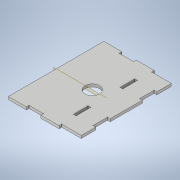
# Autodesk Inventor part: Side_two
Saved by Autodesk Inventor 2020 (Build 240168000, 168)
## iProperties
Created: 2019-12-17
Part Number: Side_two
Material: Generic
Document SubType Name: Modeling
Designer: fabfarm
Density: 1 g/cm^3
Appearance: Default
Author: fabfarm
Autodesk Inventor part; units mm, degrees
ref_plane "YZ Plane" through (0, 0, 0) normal (1, 0, 0) x (0, 1, 0)
ref_plane "XZ Plane" through (0, 0, 0) normal (0, 1, 0) x (-1, 0, 0)
ref_plane "XY Plane" through (0, 0, 0) normal (0, 0, 1) x (1, 0, 0)
sketch "Sketch1" plane through (0, 0, 0) normal (0, 1, 0) x (-1, 0, 0)
  line L0 (0, 0) -> (485, 0)
  line L1 (485, 0) -> (485, 660)
  line L2 (485, 660) -> (0, 660)
  line L3 (0, 660) -> (0, 0)
  dimension "d0" = 485
  dimension "d1" = 660
  constraints: 8 end point, 2 parallel, 1 horizontal, 1 perpendicular
  measures "d0" distance of L0.start L0.end
  measures "d1" distance of L2.end L0.start
extrude "Extrusion1" add sketch "Sketch1" along normal blind 18.55
ref_plane "Work Plane1" through (-485, 0, 330) normal (0, 0, 1) x (1, 0, 0)
sketch "Sketch4" plane through (0, 18.55, 0) normal (0, 1, 0) x (1, 0, 0)
  circle A0 centre (-235, -330) radius 50
  line L0 (97, -330) -> (-582, -330) projected
  line L1 (0, -660) -> (0, 0) projected
  point P0 (0, -641.45)
  point P1 (0, -18.55)
  dimension "d20" = 100
  dimension "d21" = 235
  constraints: 1 centre point, 1 point on line
  measures "d20" diameter of A0
  measures "d21" distance from line of L1 A0.centre
extrude "Extrusion4" cut sketch "Sketch4" against normal blind 20
sketch "Esquisse5" plane through (0, 18.55, 0) normal (0, 1, 0) x (1, 0, 0)
  line L0 (-485, -660) -> (0, -660) projected
  line L1 (-360.1, -660) -> (-259.9, -660)
  line L2 (-259.9, -660) -> (-259.9, -641.45)
  line L3 (-259.9, -641.45) -> (-360.1, -641.45)
  line L4 (-360.1, -641.45) -> (-360.1, -660)
  line L5 (0, 0) -> (-485, 0) projected
  line L6 (-360.1, 0) -> (-259.9, 0)
  line L7 (-259.9, 0) -> (-259.9, -18.55)
  line L8 (-259.9, -18.55) -> (-360.1, -18.55)
  line L9 (-360.1, -18.55) -> (-360.1, 0)
  line L10 (-485, 0) -> (-485, -660) projected
  line L11 (0, -660) -> (0, 0) projected
  point P0 (-259.9, -660)
  dimension "d24" = 100.2
  dimension "d25" = 124.9
  dimension "d26" = 18.55
  dimension "d27" = 18.55
  dimension "d28" = 259.9
  constraints: 16 end point, 4 parallel, 4 point on line, 2 horizontal, 2 perpendicular
  measures "d24" distance of L2.end L3.end
  measures "d25" distance between parallel lines of L10 L4
  measures "d26" distance of L1.end L2.end
  measures "d27" distance of L6.end L7.end
  measures "d28" distance from line of L11 L1.end
extrude "Extrusion5" cut sketch "Esquisse5" against normal blind 100 contours L4 L3 L2 L0 | L5 L7 L8 L9
sketch "Esquisse6" plane through (0, 18.55, 0) normal (0, 1, 0) x (1, 0, 0)
  line L0 (-259.9, -18.55) -> (-360.1, -18.55) projected
  circle A0 centre (-360.1, -18.55) radius 1.585
  circle A1 centre (-259.9, -18.55) radius 1.585
  line L1 (-259.9, -641.45) -> (-360.1, -641.45) projected
  circle A2 centre (-360.1, -641.45) radius 1.585
  circle A3 centre (-259.9, -641.45) radius 1.585
  point P0 (0, 0)
  dimension "d31" = 3.17
  constraints: 4 centre point, 3 equal radius, 2 coincident
  measures "d31" diameter of A3
extrude "Extrusion6" cut sketch "Esquisse6" against normal blind 100
sketch "Esquisse7" plane through (0, 18.55, 0) normal (0, 1, 0) x (1, 0, 0)
  line L0 (-134.85, -541.5) -> (-153.5, -541.5)
  line L1 (-153.5, -541.5) -> (-153.5, -441.4)
  line L2 (-153.5, -441.4) -> (-134.85, -441.4)
  line L3 (-134.85, -441.4) -> (-134.85, -541.5)
  line L4 (-134.85, -218.6) -> (-153.5, -218.6)
  line L5 (-153.5, -218.6) -> (-153.5, -118.5)
  line L6 (-153.5, -118.5) -> (-134.85, -118.5)
  line L7 (-134.85, -118.5) -> (-134.85, -218.6)
  line L8 (0, 0) -> (-259.9, 0) projected
  line L9 (-259.9, -660) -> (0, -660) projected
  line L10 (-259.9, -643.035) -> (-259.9, -660) projected
  dimension "d34" = 118.5
  dimension "d35" = 100.1
  dimension "d36" = 100.1
  dimension "d37" = 118.5
  dimension "d38" = 18.65
  dimension "d45" = 106.4
  constraints: 16 end point, 4 parallel, 2 collinear, 2 horizontal, 2 perpendicular
  measures "d34" distance between parallel lines of L8 L6
  measures "d35" distance of L4.end L5.end
  measures "d36" distance of L0.end L1.end
  measures "d37" distance between parallel lines of L9 L0
  measures "d38" distance of L1.end L2.end
  measures "d45" distance between parallel lines of L10 L1
extrude "Extrusion7" cut sketch "Esquisse7" against normal blind 20
sketch "Esquisse8" plane through (0, 18.55, 0) normal (0, 1, 0) x (1, 0, 0)
  line L0 (-153.5, -541.5) -> (-153.5, -441.4) projected
  circle A0 centre (-153.5, -541.5) radius 1.6
  circle A1 centre (-153.5, -441.4) radius 1.6
  line L1 (-153.5, -218.6) -> (-153.5, -118.5) projected
  circle A2 centre (-153.5, -218.6) radius 1.6
  circle A3 centre (-153.5, -118.5) radius 1.6
  point P0 (0, 0)
  dimension "d41" = 3.2
  constraints: 4 centre point, 3 equal radius, 2 coincident
  measures "d41" diameter of A2
extrude "Extrusion8" cut sketch "Esquisse8" against normal blind 20
sketch "Esquisse9" plane through (0, 18.55, 0) normal (0, 1, 0) x (1, 0, 0)
  line L0 (-259.9, -660) -> (0, -660) projected
  line L1 (0, -660) -> (-135, -660)
  line L2 (-135, -660) -> (-135, -641.45)
  line L3 (-135, -641.45) -> (0, -641.45)
  line L4 (0, -641.45) -> (0, -660)
  line L5 (0, 0) -> (-135, 0)
  line L6 (-135, 0) -> (-135, -18.55)
  line L7 (-135, -18.55) -> (0, -18.55)
  line L8 (0, -18.55) -> (0, 0)
  dimension "d46" = 135
  dimension "d47" = 18.55
  constraints: 16 end point, 4 parallel, 2 collinear, 2 horizontal, 2 perpendicular
  measures "d46" distance of L2.end L3.end
  measures "d47" distance of L3.end L0.end
extrude "Extrusion9" cut sketch "Esquisse9" against normal blind 20
sketch "Esquisse10" plane through (0, 18.55, 0) normal (0, 1, 0) x (1, 0, 0)
  line L0 (0, -641.45) -> (0, -18.55) projected
  line L1 (0, -541.5) -> (-18.55, -541.5)
  line L2 (-18.55, -541.5) -> (-18.55, -441.4)
  line L3 (-18.55, -441.4) -> (0, -441.4)
  line L4 (0, -441.4) -> (0, -541.5)
  line L5 (0, -218.6) -> (-18.55, -218.6)
  line L6 (-18.55, -218.6) -> (-18.55, -118.5)
  line L7 (-18.55, -118.5) -> (0, -118.5)
  line L8 (0, -118.5) -> (0, -218.6)
  line L9 (-134.85, -541.5) -> (-151.9, -541.5) projected
  line L10 (-151.9, -441.4) -> (-134.85, -441.4) projected
  line L11 (-134.85, -218.6) -> (-151.9, -218.6) projected
  line L12 (-151.9, -118.5) -> (-134.85, -118.5) projected
  point P0 (0, 0)
  point P1 (0, -441.4)
  point P2 (0, -118.5)
  dimension "d50" = 18.55
  constraints: 16 end point, 4 collinear, 4 parallel, 3 point on line, 2 horizontal, 2 perpendicular
  measures "d50" distance of L1.start L1.end
extrude "Extrusion10" cut sketch "Esquisse10" against normal blind 20
sketch "Esquisse11" plane through (0, 18.55, 0) normal (0, 1, 0) x (1, 0, 0)
  line L0 (-18.55, -541.5) -> (-18.55, -441.4) projected
  circle A0 centre (-18.55, -541.5) radius 1.6
  circle A1 centre (-18.55, -441.4) radius 1.6
  circle A2 centre (-134.85, -541.5) radius 1.6
  circle A3 centre (-134.85, -441.4) radius 1.6
  line L1 (-135, -641.45) -> (0, -641.45) projected
  circle A4 centre (-135, -641.45) radius 1.6
  line L2 (-134.85, -218.6) -> (-151.9, -218.6) projected
  circle A5 centre (-134.85, -218.6) radius 1.6
  circle A6 centre (-18.55, -218.6) radius 1.6
  line L3 (-134.85, -218.6) -> (-134.85, -118.5) projected
  circle A7 centre (-134.85, -118.5) radius 1.6
  circle A8 centre (-18.55, -118.5) radius 1.6
  line L4 (0, -18.55) -> (-135, -18.55) projected
  circle A9 centre (-135, -18.55) radius 1.6
  point P0 (0, 0)
  dimension "d53" = 3.2
  constraints: 10 centre point, 9 equal radius, 5 coincident
  measures "d53" diameter of A3
extrude "Extrusion11" cut sketch "Esquisse11" against normal blind 20
body "Solid1"
